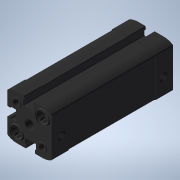
# Autodesk Inventor part: 537123 ADNGF-12-40-P-A---(Z)
Saved by Autodesk Inventor 2021 (Build 250183000, 183)
## iProperties
Created: 2025-06-05
Part Number: 537123 ADNGF-12-40-P-A---(Z)
Material: Generic
Catalog Web Link: www.cadenas.de
Description: ADN-(Z(mm))-Compact cylinder - Z
Vendor: FESTO
Document SubType Name: Modeling
Designer: psAdmin
Manufacturer: FESTO
Mass: 35.9868 g
Surface Area: 194.795 cm^2
Volume: 35.9868 cm^3
Density: 1 g/cm^3
Appearance: PSOLRGB-175-175-175
Category: PARTsolutions
Company: FESTO
Title: 537123 ADNGF-12-40-P-A---(Z)
Author: Cadenas PARTsolutions
Comments: Compact cylinder - Z
PSOL_IDENT_0: {$CADENAS_DATA/23d-libs/festo/parts/a/adngf/parts/adngf_zr.prj},215 {VTYP=3D},{NB=537123 ADNGF-12-40
PSOL_IDENT_1: -P-A---(Z)},{LINA=537123 ADNGF-12-40-P-A---(Z)},{NN=ADN-(Z(mm))},{DATE=02.05.2022 13:23:46},{GEOMDAT
PSOL_IDENT_2: E=06.10.2021 08:16:00},{VERSION=},{LINEID=5510},{WBVAR=HUB,S2S20},{WBNUMERIC=HUB}  {NB=537123 ADNGF-
PSOL_IDENT_3: 12-40-P-A---(Z)},{LINA=537123 ADNGF-12-40-P-A---(Z)},{KT=ADNGF-12},{TNR=537123},{AUSF=ADNGF-12},{KDM=
PSOL_IDENT_4: 12},{BG=17.000},{VERS=1},{HUB=40.00000},{HUB1=1.000},{HUB2=200.000},{ED=P-A},{Q=-},{S2S20=-},{S1=-},
PSOL_IDENT_5: {R8=-},{TT=-},{A=10.000},{A1=0.000},{AF=8.000},{AF1=0.000},{AF2=8.000},{AF3=0.000},{B=0.000},{B1=0.0
PSOL_IDENT_6: 00},{BG1=0.000},{D1=9.000},{D2=6.000},{D3=32.000},{D4=0.000},{D5=4.000},{D6=M3},{D7=3.000},{D8=0.000
PSOL_IDENT_7: },{D9=0.000},{E=27.500},{EE=M5},{EEN=5.000},{EE1=-},{J=10.500},{J1=2.000},{J11=2},{J2=0.000},{KF=4-4
PSOL_IDENT_8: 8 UNF-2B},{KF1=-},{KF2=4-45 UNF-2B},{KF3=-},{KK=10-32 UNF-2A},{KK1=-},{L1=1.500},{L2=35.000},{L3=2.1
PSOL_IDENT_9: 00},{L4=3.500},{L5=0.000},{L6=46.000},{L7=12.000},{L8=0.000},{L9=1.500},{L10=0.000},{L11=0.000},{MF=
PSOL_IDENT_10: 6.000},{MM=6.000},{MM1=0.000},{PL=6.000},{RT=M4},{RTN=4},{RTNK=3.242},{SF=3/16},{SF1=-},{SW=5.500},{
PSOL_IDENT_11: TG=16.000},{VD=0.000},{VD1=0.000},{WH=4.200},{WH1=0.000},{WL=2.700},{WL1=0.000},{Y1=0.300},{Y2=0.500
PSOL_IDENT_12: },{ZJ=39.200},{ZM=43.400},{RU=16.600},{R1=10.350},{R2=0.600},{RA=0.600},{RR=5.600},{RB1=5.400},{RB2=
PSOL_IDENT_13: 6.800},{RT1=3.400},{DSK=6.000},{MDK=5.500},{MK=3.000},{MT=1.300},{MS=2.500},{RUB=0.200},{KFN=3.000},
PSOL_IDENT_14: {KFK=2.459},{B111=9.200},{B11=1.000},{B2=5.000},{B3=8.500},{B4=3.500},{B5=3.000},{B6=6.000},{B7=17.0
PSOL_IDENT_15: 00},{B8=4.000},{B9=6.000},{B10=7.200},{W=0.400},{S=6.000},{LA=0.000},{LA1=0.000},{LA2=5.500},{LA3=7.
PSOL_IDENT_16: 000},{LA31=8.000},{LA4=0.000},{LA5=0.000},{LA6=0.000},{LA7=0.000},{LA8=0.000},{LA9=0.000},{LA10=0.00
PSOL_IDENT_17: 0},{ES=0.000},{SS=0.000},{TS=0.000},{WS=0.000},{DK=0.000},{KS=0.000},{S2N=},{D10=5.500},{D11=6.200},
PSOL_IDENT_18: {D12=0.200},{D13=4.000},{D14=0.000},{L12=15.000},{L13=4.200}
NB: 537123 ADNGF-12-40-P-A---(Z)
NN: ADN-(Z(mm))
NT: Compact cylinder - Z
NBSYN: $TNR. $AUSF.-$HUB.-$ED.$S2N.---(Z)
LINA: 537123 ADNGF-12-40-P-A---(Z)
CATALOG: Festo
TNR: 537123
AUSF: ADNGF-12
KDM: 12
BG: 17
HUB: 40
ED: P-A
Q: -
S2S20: -
S1: -
R8: -
TT: -
A: 10
A1: 0
AF: 8
AF1: 0
AF2: 8
AF3: 0
B: 0
B1: 0
BG1: 0
D1: 9
D2: 6
D3: 32
D4: 0
D5: 4
D6: M3
D7: 3
D8: 0
D9: 0
E: 27.5
EE: M5
EE1: -
J: 10.5
J1: 2
J2: 0
KF: 4-48 UNF-2B
KF1: -
KF2: 4-45 UNF-2B
KF3: -
KK: 10-32 UNF-2A
KK1: -
L1: 1.5
L2: 35
L3: 2.1
L4: 3.5
L5: 0
L6: 46
L7: 12
L8: 0
L9: 1.5
L10: 0
L11: 0
MF: 6
MM: 6
MM1: 0
PL: 6
RT: M4
RTNK: 3.242
SF: 3/16
SF1: -
SW: 5.5
TG: 16
VD: 0
VD1: 0
WH: 4.2
WH1: 0
WL: 2.7
WL1: 0
Y1: 0.3
Y2: 0.5
ZJ: 39.2
ZM: 43.4
RU: 16.6
R1: 10.35
R2: 0.6
RA: 0.6
RR: 5.6
DSK: 6
MDK: 5.5
MK: 3
MT: 1.3
MS: 2.5
RUB: 0.2
B111: 9.2
B11: 1
B2: 5
B3: 8.5
B4: 3.5
B5: 3
B6: 6
B7: 17
B8: 4
B9: 6
B10: 7.2
W: 0.4
S: 6
LA: 0
LA1: 0
LA2: 5.5
LA3: 7
LA31: 8
LA4: 0
LA5: 0
LA6: 0
LA7: 0
LA8: 0
LA9: 0
LA10: 0
ES: 0
SS: 0
TS: 0
WS: 0
DK: 0
KS: 0
D10: 5.5
D11: 6.2
D12: 0.2
D13: 4
D14: 0
L12: 15
L13: 4.2
SUPPLIER: FESTO
ARTICLENO: 537123 ADNGF-12-40-P-A---(Z)
BOMINFO: 537123 ADNGF-12-40-P-A---(Z)
CREATOR: CADENAS GmbH
Autodesk Inventor part; units mm, degrees
sketch "Sketch_26" plane through (0, 0, 0) normal (0, 0, 1) x (1, 0, 0)
  line L0 (-13.75, -2.5) -> (-13.75, -11.5793)
  arc A0 (-13.75, -11.5793) -> (-13.3272, -12.3141) centre (-12.9, -11.5793) ccw
  arc A1 (-13.3272, -12.3141) -> (-8, -13.75) centre (-8, -3.15) ccw
  line L1 (-8, -13.75) -> (-2.5, -13.75)
  arc A2 (-2.5, -13.75) -> (-2.1, -13.35) centre (-2.5, -13.35) ccw
  line L2 (-2.1, -13.35) -> (-2.1, -11.9)
  arc A3 (-2.1, -11.9) -> (-2.3, -11.7) centre (-2.3, -11.9) ccw
  line L3 (-2.3, -11.7) -> (-2.6, -11.7)
  arc A4 (-2.8, -11.5) -> (-2.6, -11.7) centre (-2.6, -11.5) ccw
  line L4 (-2.8, -11.5) -> (-2.8, -8.7)
  arc A5 (-2.4, -8.3) -> (-2.8, -8.7) centre (-2.4, -8.7) ccw
  line L5 (-2.4, -8.3) -> (3.6, -8.3)
  arc A6 (4, -8.7) -> (3.6, -8.3) centre (3.6, -8.7) ccw
  line L6 (4, -8.7) -> (4, -11.5)
  arc A7 (3.8, -11.7) -> (4, -11.5) centre (3.8, -11.5) ccw
  line L7 (3.8, -11.7) -> (3.5, -11.7)
  arc A8 (3.5, -11.7) -> (3.3, -11.9) centre (3.5, -11.9) ccw
  line L8 (3.3, -11.9) -> (3.3, -13.35)
  arc A9 (3.3, -13.35) -> (3.7, -13.75) centre (3.7, -13.35) ccw
  line L9 (3.7, -13.75) -> (8, -13.75)
  arc A10 (8, -13.75) -> (13.3272, -12.3141) centre (8, -3.15) ccw
  arc A11 (13.3272, -12.3141) -> (13.75, -11.5793) centre (12.9, -11.5793) ccw
  line L10 (13.75, -11.5793) -> (13.75, 11.5793)
  arc A12 (13.75, 11.5793) -> (13.3272, 12.3141) centre (12.9, 11.5793) ccw
  arc A13 (13.3272, 12.3141) -> (8, 13.75) centre (8, 3.15) ccw
  line L11 (8, 13.75) -> (2.5, 13.75)
  arc A14 (2.5, 13.75) -> (2.1, 13.35) centre (2.5, 13.35) ccw
  line L12 (2.1, 13.35) -> (2.1, 11.9)
  arc A15 (2.1, 11.9) -> (2.3, 11.7) centre (2.3, 11.9) ccw
  line L13 (2.3, 11.7) -> (2.6, 11.7)
  arc A16 (2.8, 11.5) -> (2.6, 11.7) centre (2.6, 11.5) ccw
  line L14 (2.8, 11.5) -> (2.8, 8.7)
  arc A17 (2.4, 8.3) -> (2.8, 8.7) centre (2.4, 8.7) ccw
  line L15 (2.4, 8.3) -> (-3.6, 8.3)
  arc A18 (-4, 8.7) -> (-3.6, 8.3) centre (-3.6, 8.7) ccw
  line L16 (-4, 8.7) -> (-4, 11.5)
  arc A19 (-3.8, 11.7) -> (-4, 11.5) centre (-3.8, 11.5) ccw
  line L17 (-3.8, 11.7) -> (-3.5, 11.7)
  arc A20 (-3.5, 11.7) -> (-3.3, 11.9) centre (-3.5, 11.9) ccw
  line L18 (-3.3, 11.9) -> (-3.3, 13.35)
  arc A21 (-3.3, 13.35) -> (-3.7, 13.75) centre (-3.7, 13.35) ccw
  line L19 (-3.7, 13.75) -> (-8, 13.75)
  arc A22 (-8, 13.75) -> (-13.3272, 12.3141) centre (-8, 3.15) ccw
  arc A23 (-13.3272, 12.3141) -> (-13.75, 11.5793) centre (-12.9, 11.5793) ccw
  line L20 (-13.75, 11.5793) -> (-13.75, 3.7)
  arc A24 (-13.75, 3.7) -> (-13.35, 3.3) centre (-13.35, 3.7) ccw
  line L21 (-13.35, 3.3) -> (-11.9, 3.3)
  arc A25 (-11.9, 3.3) -> (-11.7, 3.5) centre (-11.9, 3.5) ccw
  line L22 (-11.7, 3.5) -> (-11.7, 3.8)
  arc A26 (-11.5, 4) -> (-11.7, 3.8) centre (-11.5, 3.8) ccw
  line L23 (-11.5, 4) -> (-8.7, 4)
  arc A27 (-8.3, 3.6) -> (-8.7, 4) centre (-8.7, 3.6) ccw
  line L24 (-8.3, 3.6) -> (-8.3, -2.4)
  arc A28 (-8.7, -2.8) -> (-8.3, -2.4) centre (-8.7, -2.4) ccw
  line L25 (-8.7, -2.8) -> (-11.5, -2.8)
  arc A29 (-11.7, -2.6) -> (-11.5, -2.8) centre (-11.5, -2.6) ccw
  line L26 (-11.7, -2.6) -> (-11.7, -2.3)
  arc A30 (-11.7, -2.3) -> (-11.9, -2.1) centre (-11.9, -2.3) ccw
  line L27 (-11.9, -2.1) -> (-13.35, -2.1)
  arc A31 (-13.35, -2.1) -> (-13.75, -2.5) centre (-13.35, -2.5) ccw
  constraints: 64 point on circle, 56 end point, 32 centre point
extrude "Extrusion1" add sketch "Sketch_26" against normal blind 75
sketch "Sketch_112" plane through (0, 0, -10.5) normal (0, 0, 1) x (1, 0, 0)
  line L0 (-27.5, -27.5) -> (27.5, -27.5)
  line L1 (27.5, -27.5) -> (27.5, 27.5)
  line L2 (27.5, 27.5) -> (-27.5, 27.5)
  line L3 (-27.5, 27.5) -> (-27.5, -27.5)
  line L4 (-13.5, -2.5) -> (-13.5, -11.3293)
  arc A0 (-13.5, -11.3293) -> (-13.0772, -12.0641) centre (-12.65, -11.3293) ccw
  arc A1 (-13.0772, -12.0641) -> (-7.75, -13.5) centre (-7.75, -2.9) ccw
  line L5 (-7.75, -13.5) -> (-2.5, -13.5)
  arc A2 (-2.5, -13.5) -> (-2.1, -13.1) centre (-2.5, -13.1) ccw
  line L6 (-2.1, -13.1) -> (-2.1, -11.9)
  arc A3 (-2.1, -11.9) -> (-2.3, -11.7) centre (-2.3, -11.9) ccw
  line L7 (-2.3, -11.7) -> (-2.6, -11.7)
  arc A4 (-2.8, -11.5) -> (-2.6, -11.7) centre (-2.6, -11.5) ccw
  line L8 (-2.8, -11.5) -> (-2.8, -8.7)
  arc A5 (-2.4, -8.3) -> (-2.8, -8.7) centre (-2.4, -8.7) ccw
  line L9 (-2.4, -8.3) -> (3.6, -8.3)
  arc A6 (4, -8.7) -> (3.6, -8.3) centre (3.6, -8.7) ccw
  line L10 (4, -8.7) -> (4, -11.5)
  arc A7 (3.8, -11.7) -> (4, -11.5) centre (3.8, -11.5) ccw
  line L11 (3.8, -11.7) -> (3.5, -11.7)
  arc A8 (3.5, -11.7) -> (3.3, -11.9) centre (3.5, -11.9) ccw
  line L12 (3.3, -11.9) -> (3.3, -13.1)
  arc A9 (3.3, -13.1) -> (3.7, -13.5) centre (3.7, -13.1) ccw
  line L13 (3.7, -13.5) -> (7.75, -13.5)
  arc A10 (7.75, -13.5) -> (13.0772, -12.0641) centre (7.75, -2.9) ccw
  arc A11 (13.0772, -12.0641) -> (13.5, -11.3293) centre (12.65, -11.3293) ccw
  line L14 (13.5, -11.3293) -> (13.5, 11.3293)
  arc A12 (13.5, 11.3293) -> (13.0772, 12.0641) centre (12.65, 11.3293) ccw
  arc A13 (13.0772, 12.0641) -> (7.75, 13.5) centre (7.75, 2.9) ccw
  line L15 (7.75, 13.5) -> (2.5, 13.5)
  arc A14 (2.5, 13.5) -> (2.1, 13.1) centre (2.5, 13.1) ccw
  line L16 (2.1, 13.1) -> (2.1, 11.9)
  arc A15 (2.1, 11.9) -> (2.3, 11.7) centre (2.3, 11.9) ccw
  line L17 (2.3, 11.7) -> (2.6, 11.7)
  arc A16 (2.8, 11.5) -> (2.6, 11.7) centre (2.6, 11.5) ccw
  line L18 (2.8, 11.5) -> (2.8, 8.7)
  arc A17 (2.4, 8.3) -> (2.8, 8.7) centre (2.4, 8.7) ccw
  line L19 (2.4, 8.3) -> (-3.6, 8.3)
  arc A18 (-4, 8.7) -> (-3.6, 8.3) centre (-3.6, 8.7) ccw
  line L20 (-4, 8.7) -> (-4, 11.5)
  arc A19 (-3.8, 11.7) -> (-4, 11.5) centre (-3.8, 11.5) ccw
  line L21 (-3.8, 11.7) -> (-3.5, 11.7)
  arc A20 (-3.5, 11.7) -> (-3.3, 11.9) centre (-3.5, 11.9) ccw
  line L22 (-3.3, 11.9) -> (-3.3, 13.1)
  arc A21 (-3.3, 13.1) -> (-3.7, 13.5) centre (-3.7, 13.1) ccw
  line L23 (-3.7, 13.5) -> (-7.75, 13.5)
  arc A22 (-7.75, 13.5) -> (-13.0772, 12.0641) centre (-7.75, 2.9) ccw
  arc A23 (-13.0772, 12.0641) -> (-13.5, 11.3293) centre (-12.65, 11.3293) ccw
  line L24 (-13.5, 11.3293) -> (-13.5, 3.7)
  arc A24 (-13.5, 3.7) -> (-13.1, 3.3) centre (-13.1, 3.7) ccw
  line L25 (-13.1, 3.3) -> (-11.9, 3.3)
  arc A25 (-11.9, 3.3) -> (-11.7, 3.5) centre (-11.9, 3.5) ccw
  line L26 (-11.7, 3.5) -> (-11.7, 3.8)
  arc A26 (-11.5, 4) -> (-11.7, 3.8) centre (-11.5, 3.8) ccw
  line L27 (-11.5, 4) -> (-8.7, 4)
  arc A27 (-8.3, 3.6) -> (-8.7, 4) centre (-8.7, 3.6) ccw
  line L28 (-8.3, 3.6) -> (-8.3, -2.4)
  arc A28 (-8.7, -2.8) -> (-8.3, -2.4) centre (-8.7, -2.4) ccw
  line L29 (-8.7, -2.8) -> (-11.5, -2.8)
  arc A29 (-11.7, -2.6) -> (-11.5, -2.8) centre (-11.5, -2.6) ccw
  line L30 (-11.7, -2.6) -> (-11.7, -2.3)
  arc A30 (-11.7, -2.3) -> (-11.9, -2.1) centre (-11.9, -2.3) ccw
  line L31 (-11.9, -2.1) -> (-13.1, -2.1)
  arc A31 (-13.1, -2.1) -> (-13.5, -2.5) centre (-13.1, -2.5) ccw
  constraints: 64 end point, 64 point on circle, 32 centre point
extrude "Extrusion2" cut sketch "Sketch_112" against normal blind 54
sketch "Sketch3" plane through (13.75, -11.5793, 0) normal (1, 0, 0) x (0, 0, -1)
  point P0 (6, 9.5793)
hole "Hole1" at (13.75, -2, -6) direction (-1, 0, 0) diameter 4.134 depth 7 countersink diameter 5 countersink angle 90 thread size "M5x0.8" class "6H" standard "ISO Metric profile"
sketch "Sketch4" plane through (13.75, -11.5793, -75) normal (1, 0, 0) x (0, 0, -1)
  point P0 (-6, 9.5793)
hole "Hole2" at (13.75, -2, -69) direction (-1, 0, 0) diameter 4.134 depth 8 countersink diameter 5 countersink angle 90 thread size "M5x0.8" class "6H" standard "ISO Metric profile"
sketch "Skizze_5" plane through (0, 0, 0) normal (1, 0, 0) x (0, 1, 0)
  line L0 (0, -63) -> (0, 1)
  line L1 (0, 1) -> (3, 1)
  line L2 (3, 1) -> (3, -20)
  line L3 (3, -20) -> (6, -20)
  line L4 (6, -20) -> (6, -63)
  line L5 (6, -63) -> (0, -63)
  line L6 (0, -63) -> (0, 1)
  constraints: 14 end point
revolve "Revolution1" cut sketch "Skizze_5" angle 360 about axis through (0, 0, -63) along (0, 0, -1)
sketch "Sketch6" plane through (0, 0, -75) normal (0, 0, -1) x (-1, 0, 0)
  point P0 (0, 0)
hole "Hole3" at (0, 0, -75) direction (0, 0, 1) diameter 9 depth 2.1
sketch "Sketch7" plane through (0, 0, 0) normal (0, 0, 1) x (1, 0, 0)
  point P0 (8, 8)
hole "Hole4" at (8, 8, 0) direction (0, 0, -1) diameter 6 depth 17 counterbore diameter 9.2 counterbore depth 5
sketch "Sketch_27" plane through (8, 0, 0) normal (1, 0, 0) x (0, 0, -1)
  line L0 (17, 8) -> (0, 8)
  line L1 (0, 11.6) -> (1.0392, 11)
  line L2 (1.0392, 11) -> (3.5, 11)
  line L3 (3.5, 11) -> (3.5, 10)
  line L4 (3.5, 10) -> (3.879, 9.621)
  line L5 (3.879, 9.621) -> (17, 9.621)
  line L6 (17, 9.621) -> (17, 12)
  line L7 (17, 12) -> (5, 12)
  line L8 (5, 12) -> (5, 12.25)
  line L9 (5, 12.25) -> (0.4, 12.25)
  line L10 (0.4, 12.25) -> (0, 11.85)
  line L11 (0, 11.85) -> (0, 11.6)
  constraints: 24 end point
revolve "Revolution2" add sketch "Sketch_27" angle 360 about axis through (8, 8, -17) along (0, 0, -1)
thread "Thread1" size "M4x0.7" class "6H" standard "ISO Metric profile" full length
sketch "Sketch9" plane through (0, 0, -75) normal (0, 0, -1) x (-1, 0, 0)
  point P0 (-8, 8)
hole "Hole5" at (8, 8, -75) direction (0, 0, 1) diameter 6 depth 17 counterbore diameter 9.2 counterbore depth 5
sketch "Sketch10" plane through (8, 8, -58) normal (0, 0, -1) x (-1, 0, 0)
  point P0 (0, 0)
hole "Hole6" at (8, 8, -58) direction (0, 0, 1) diameter 5.6 depth 41
sketch "Sketch_28" plane through (8, 0, 0) normal (1, 0, 0) x (0, 0, -1)
  line L0 (75, 8) -> (58, 8)
  line L1 (58, 12) -> (58, 9.621)
  line L2 (58, 9.621) -> (71.121, 9.621)
  line L3 (71.121, 9.621) -> (71.5, 10)
  line L4 (71.5, 10) -> (71.5, 11)
  line L5 (71.5, 11) -> (73.9608, 11)
  line L6 (73.9608, 11) -> (75, 11.6)
  line L7 (75, 11.6) -> (75, 11.85)
  line L8 (75, 11.85) -> (74.6, 12.25)
  line L9 (74.6, 12.25) -> (70, 12.25)
  line L10 (70, 12.25) -> (70, 12)
  line L11 (70, 12) -> (58, 12)
  constraints: 24 end point
revolve "Revolution3" add sketch "Sketch_28" angle 360 about axis through (8, 8, -75) along (0, 0, -1)
thread "Thread2" size "M4x0.7" class "6H" standard "ISO Metric profile" full length
sketch "Sketch12" plane through (0, 0, 0) normal (0, 0, 1) x (1, 0, 0)
  point P0 (-8, -8)
hole "Hole7" at (-8, -8, 0) direction (0, 0, -1) diameter 6 depth 17 counterbore diameter 9.2 counterbore depth 5
sketch "Sketch13" plane through (0, 0, -75) normal (0, 0, -1) x (-1, 0, 0)
  point P0 (8, -8)
hole "Hole8" at (-8, -8, -75) direction (0, 0, 1) diameter 6 depth 17 counterbore diameter 9.2 counterbore depth 5
sketch "Sketch_29" plane through (-8, 0, 0) normal (1, 0, 0) x (0, 0, -1)
  line L0 (17, -8) -> (0, -8)
  line L1 (0, -4.4) -> (1.0392, -5)
  line L2 (1.0392, -5) -> (3.5, -5)
  line L3 (3.5, -5) -> (3.5, -6)
  line L4 (3.5, -6) -> (3.879, -6.379)
  line L5 (3.879, -6.379) -> (17, -6.379)
  line L6 (17, -6.379) -> (17, -4)
  line L7 (17, -4) -> (5, -4)
  line L8 (5, -4) -> (5, -3.75)
  line L9 (5, -3.75) -> (0.4, -3.75)
  line L10 (0.4, -3.75) -> (0, -4.15)
  line L11 (0, -4.15) -> (0, -4.4)
  constraints: 24 end point
revolve "Revolution4" add sketch "Sketch_29" angle 360 about axis through (-8, -8, -17) along (0, 0, -1)
thread "Thread3" size "M4x0.7" class "6H" standard "ISO Metric profile" full length
sketch "Sketch_30" plane through (-8, 0, 0) normal (1, 0, 0) x (0, 0, -1)
  line L0 (75, -8) -> (58, -8)
  line L1 (58, -4) -> (58, -6.379)
  line L2 (58, -6.379) -> (71.121, -6.379)
  line L3 (71.121, -6.379) -> (71.5, -6)
  line L4 (71.5, -6) -> (71.5, -5)
  line L5 (71.5, -5) -> (73.9608, -5)
  line L6 (73.9608, -5) -> (75, -4.4)
  line L7 (75, -4.4) -> (75, -4.15)
  line L8 (75, -4.15) -> (74.6, -3.75)
  line L9 (74.6, -3.75) -> (70, -3.75)
  line L10 (70, -3.75) -> (70, -4)
  line L11 (70, -4) -> (58, -4)
  constraints: 24 end point
revolve "Revolution5" add sketch "Sketch_30" angle 360 about axis through (-8, -8, -75) along (0, 0, -1)
thread "Thread4" size "M4x0.7" class "6H" standard "ISO Metric profile" full length
sketch "Sketch16" plane through (0, 0, 0) normal (0, 0, 1) x (1, 0, 0)
  point P0 (8, -8)
hole "Hole9" at (8, -8, 0) direction (0, 0, -1) diameter 4 depth 58 counterbore diameter 5.5 counterbore depth 10.5
sketch "Sketch_14" plane through (8, 0, 0) normal (1, 0, 0) x (0, 0, -1)
  line L0 (14.7, -8) -> (-0.3, -8)
  line L1 (-0.3, -6) -> (14.7, -6)
  line L2 (14.7, -6) -> (14.7, -4.9)
  line L3 (14.7, -4.9) -> (10.5, -4.9)
  line L4 (10.5, -4.9) -> (10.5, -5.25)
  line L5 (10.5, -5.25) -> (-0.1, -5.25)
  line L6 (-0.1, -5.25) -> (-0.3, -5.3655)
  line L7 (-0.3, -5.3655) -> (-0.3, -6)
  constraints: 16 end point
revolve "Revolution6" add sketch "Sketch_14" angle 360 about axis through (8, -8, -14.7) along (0, 0, -1)
sketch "Sketch_3" plane through (8, 0, 0) normal (1, 0, 0) x (0, 0, -1)
  line L0 (75.1, -8) -> (64.5, -8)
  line L1 (64.5, -8) -> (64.5, -6.379)
  line L2 (64.5, -6.379) -> (71.121, -6.379)
  line L3 (71.121, -6.379) -> (71.5, -6)
  line L4 (71.5, -6) -> (71.5, -5)
  line L5 (71.5, -5) -> (75.1, -5)
  line L6 (75.1, -5) -> (75.1, -8)
  line L7 (75.1, -8) -> (64.5, -8)
  constraints: 16 end point
revolve "Revolution7" cut sketch "Sketch_3" angle 360 about axis through (8, -8, -75.1) along (0, 0, -1)
thread "Thread5" size "M4x0.7" class "6H" standard "ISO Metric profile" full length
sketch "Sketch19" plane through (8, -8, -64.5) normal (0, 0, -1) x (-1, 0, 0)
  point P0 (0, 0)
hole "Hole10" at (8, -8, -64.5) direction (0, 0, 1) diameter 4 depth 47.5
sketch "Sketch20" plane through (0, 0, 0) normal (0, 0, 1) x (1, 0, 0)
  point P0 (-8, 8)
hole "Hole11" at (-8, 8, 0) direction (0, 0, -1) diameter 4 depth 58 counterbore diameter 5.5 counterbore depth 10.5
sketch "Sketch_15" plane through (-8, 0, 0) normal (1, 0, 0) x (0, 0, -1)
  line L0 (14.7, 8) -> (-0.3, 8)
  line L1 (-0.3, 10) -> (14.7, 10)
  line L2 (14.7, 10) -> (14.7, 11.1)
  line L3 (14.7, 11.1) -> (10.5, 11.1)
  line L4 (10.5, 11.1) -> (10.5, 10.75)
  line L5 (10.5, 10.75) -> (-0.1, 10.75)
  line L6 (-0.1, 10.75) -> (-0.3, 10.6345)
  line L7 (-0.3, 10.6345) -> (-0.3, 10)
  constraints: 16 end point
revolve "Revolution8" add sketch "Sketch_15" angle 360 about axis through (-8, 8, -14.7) along (0, 0, -1)
sketch "Sketch_4" plane through (-8, 0, 0) normal (1, 0, 0) x (0, 0, -1)
  line L0 (75.1, 8) -> (64.5, 8)
  line L1 (64.5, 8) -> (64.5, 9.621)
  line L2 (64.5, 9.621) -> (71.121, 9.621)
  line L3 (71.121, 9.621) -> (71.5, 10)
  line L4 (71.5, 10) -> (71.5, 11)
  line L5 (71.5, 11) -> (75.1, 11)
  line L6 (75.1, 11) -> (75.1, 8)
  line L7 (75.1, 8) -> (64.5, 8)
  constraints: 16 end point
revolve "Revolution9" cut sketch "Sketch_4" angle 360 about axis through (-8, 8, -75.1) along (0, 0, -1)
thread "Thread6" size "M4x0.7" class "6H" standard "ISO Metric profile" full length
sketch "Sketch23" plane through (-8, 8, -64.5) normal (0, 0, -1) x (-1, 0, 0)
  point P0 (0, 0)
hole "Hole12" at (-8, 8, -64.5) direction (0, 0, 1) diameter 4 depth 47.5
sketch "Sketch24" plane through (-8, -8, -58) normal (0, 0, -1) x (-1, 0, 0)
  point P0 (0, 0)
hole "Hole13" at (-8, -8, -58) direction (0, 0, 1) diameter 5.6 depth 41
sketch "Sketch_8" plane through (0, 0, 0) normal (0, 0, 1) x (1, 0, 0)
  line L0 (-11.4641, -8) -> (-11, -8.8038)
  line L1 (-11, -8.8038) -> (-11, -9.7321)
  line L2 (-11, -9.7321) -> (-10.1962, -10.1962)
  line L3 (-10.1962, -10.1962) -> (-9.7321, -11)
  line L4 (-9.7321, -11) -> (-8.8038, -11)
  line L5 (-8.8038, -11) -> (-8, -11.4641)
  line L6 (-8, -11.4641) -> (-7.1962, -11)
  line L7 (-7.1962, -11) -> (-6.2679, -11)
  line L8 (-6.2679, -11) -> (-5.8038, -10.1962)
  line L9 (-5.8038, -10.1962) -> (-5, -9.7321)
  line L10 (-5, -9.7321) -> (-5, -8.8038)
  line L11 (-5, -8.8038) -> (-4.5359, -8)
  line L12 (-4.5359, -8) -> (-5, -7.1962)
  line L13 (-5, -7.1962) -> (-5, -6.2679)
  line L14 (-5, -6.2679) -> (-5.8038, -5.8038)
  line L15 (-5.8038, -5.8038) -> (-6.2679, -5)
  line L16 (-6.2679, -5) -> (-7.1962, -5)
  line L17 (-7.1962, -5) -> (-8, -4.5359)
  line L18 (-8, -4.5359) -> (-8.8038, -5)
  line L19 (-8.8038, -5) -> (-9.7321, -5)
  line L20 (-9.7321, -5) -> (-10.1962, -5.8038)
  line L21 (-10.1962, -5.8038) -> (-11, -6.2679)
  line L22 (-11, -6.2679) -> (-11, -7.1962)
  line L23 (-11, -7.1962) -> (-11.4641, -8)
  constraints: 48 end point
extrude "Extrusion3" cut sketch "Sketch_8" against normal blind 3
sketch "Sketch_7" plane through (0, 0, 0) normal (0, 0, 1) x (1, 0, 0)
  line L0 (4.5359, 8) -> (5, 7.1962)
  line L1 (5, 7.1962) -> (5, 6.2679)
  line L2 (5, 6.2679) -> (5.8038, 5.8038)
  line L3 (5.8038, 5.8038) -> (6.2679, 5)
  line L4 (6.2679, 5) -> (7.1962, 5)
  line L5 (7.1962, 5) -> (8, 4.5359)
  line L6 (8, 4.5359) -> (8.8038, 5)
  line L7 (8.8038, 5) -> (9.7321, 5)
  line L8 (9.7321, 5) -> (10.1962, 5.8038)
  line L9 (10.1962, 5.8038) -> (11, 6.2679)
  line L10 (11, 6.2679) -> (11, 7.1962)
  line L11 (11, 7.1962) -> (11.4641, 8)
  line L12 (11.4641, 8) -> (11, 8.8038)
  line L13 (11, 8.8038) -> (11, 9.7321)
  line L14 (11, 9.7321) -> (10.1962, 10.1962)
  line L15 (10.1962, 10.1962) -> (9.7321, 11)
  line L16 (9.7321, 11) -> (8.8038, 11)
  line L17 (8.8038, 11) -> (8, 11.4641)
  line L18 (8, 11.4641) -> (7.1962, 11)
  line L19 (7.1962, 11) -> (6.2679, 11)
  line L20 (6.2679, 11) -> (5.8038, 10.1962)
  line L21 (5.8038, 10.1962) -> (5, 9.7321)
  line L22 (5, 9.7321) -> (5, 8.8038)
  line L23 (5, 8.8038) -> (4.5359, 8)
  constraints: 48 end point
extrude "Extrusion4" cut sketch "Sketch_7" against normal blind 3
sketch "Sketch_9" plane through (0, 0, -75) normal (0, 0, 1) x (1, 0, 0)
  line L0 (-11.4641, -8) -> (-11, -8.8038)
  line L1 (-11, -8.8038) -> (-11, -9.7321)
  line L2 (-11, -9.7321) -> (-10.1962, -10.1962)
  line L3 (-10.1962, -10.1962) -> (-9.7321, -11)
  line L4 (-9.7321, -11) -> (-8.8038, -11)
  line L5 (-8.8038, -11) -> (-8, -11.4641)
  line L6 (-8, -11.4641) -> (-7.1962, -11)
  line L7 (-7.1962, -11) -> (-6.2679, -11)
  line L8 (-6.2679, -11) -> (-5.8038, -10.1962)
  line L9 (-5.8038, -10.1962) -> (-5, -9.7321)
  line L10 (-5, -9.7321) -> (-5, -8.8038)
  line L11 (-5, -8.8038) -> (-4.5359, -8)
  line L12 (-4.5359, -8) -> (-5, -7.1962)
  line L13 (-5, -7.1962) -> (-5, -6.2679)
  line L14 (-5, -6.2679) -> (-5.8038, -5.8038)
  line L15 (-5.8038, -5.8038) -> (-6.2679, -5)
  line L16 (-6.2679, -5) -> (-7.1962, -5)
  line L17 (-7.1962, -5) -> (-8, -4.5359)
  line L18 (-8, -4.5359) -> (-8.8038, -5)
  line L19 (-8.8038, -5) -> (-9.7321, -5)
  line L20 (-9.7321, -5) -> (-10.1962, -5.8038)
  line L21 (-10.1962, -5.8038) -> (-11, -6.2679)
  line L22 (-11, -6.2679) -> (-11, -7.1962)
  line L23 (-11, -7.1962) -> (-11.4641, -8)
  constraints: 48 end point
extrude "Extrusion5" cut sketch "Sketch_9" along normal blind 3
sketch "Sketch_10" plane through (0, 0, -75) normal (0, 0, 1) x (1, 0, 0)
  line L0 (4.5359, 8) -> (5, 7.1962)
  line L1 (5, 7.1962) -> (5, 6.2679)
  line L2 (5, 6.2679) -> (5.8038, 5.8038)
  line L3 (5.8038, 5.8038) -> (6.2679, 5)
  line L4 (6.2679, 5) -> (7.1962, 5)
  line L5 (7.1962, 5) -> (8, 4.5359)
  line L6 (8, 4.5359) -> (8.8038, 5)
  line L7 (8.8038, 5) -> (9.7321, 5)
  line L8 (9.7321, 5) -> (10.1962, 5.8038)
  line L9 (10.1962, 5.8038) -> (11, 6.2679)
  line L10 (11, 6.2679) -> (11, 7.1962)
  line L11 (11, 7.1962) -> (11.4641, 8)
  line L12 (11.4641, 8) -> (11, 8.8038)
  line L13 (11, 8.8038) -> (11, 9.7321)
  line L14 (11, 9.7321) -> (10.1962, 10.1962)
  line L15 (10.1962, 10.1962) -> (9.7321, 11)
  line L16 (9.7321, 11) -> (8.8038, 11)
  line L17 (8.8038, 11) -> (8, 11.4641)
  line L18 (8, 11.4641) -> (7.1962, 11)
  line L19 (7.1962, 11) -> (6.2679, 11)
  line L20 (6.2679, 11) -> (5.8038, 10.1962)
  line L21 (5.8038, 10.1962) -> (5, 9.7321)
  line L22 (5, 9.7321) -> (5, 8.8038)
  line L23 (5, 8.8038) -> (4.5359, 8)
  constraints: 48 end point
extrude "Extrusion6" cut sketch "Sketch_10" along normal blind 3
ref_plane "CYLINDER_XY" through (0, 0, -63) normal (0, 0, 1) x (1, 0, 0)
ref_plane "CYLINDER_YZ" through (0, 0, -63) normal (1, 0, 0) x (0, 1, 0)
ref_plane "CYLINDER_ZX" through (0, 0, -63) normal (0, 1, 0) x (0, 0, 1)
ref_plane "QS_HINTEN_XY" through (13.75, -2, -69) normal (1, 0, 0) x (0, 0, -1)
ref_plane "QS_HINTEN_YZ" through (13.75, -2, -69) normal (0, 0, -1) x (0, 1, 0)
ref_plane "QS_HINTEN_ZX" through (13.75, -2, -69) normal (0, 1, 0) x (1, 0, 0)
ref_plane "QS_VORNE_XY" through (13.75, -2, -6) normal (1, 0, 0) x (0, 0, -1)
ref_plane "QS_VORNE_YZ" through (13.75, -2, -6) normal (0, 0, -1) x (0, 1, 0)
ref_plane "QS_VORNE_ZX" through (13.75, -2, -6) normal (0, 1, 0) x (1, 0, 0)
ref_plane "TO_DUMMY_XY" through (0, 0, 0) normal (0, 0, 1) x (1, 0, 0)
ref_plane "TO_DUMMY_YZ" through (0, 0, 0) normal (1, 0, 0) x (0, 1, 0)
ref_plane "TO_DUMMY_ZX" through (0, 0, 0) normal (0, 1, 0) x (0, 0, 1)
ref_plane "ZUBEHOER_HINTEN_XY" through (0, 0, -75) normal (0, 0, 1) x (1, 0, 0)
ref_plane "ZUBEHOER_HINTEN_YZ" through (0, 0, -75) normal (1, 0, 0) x (0, 1, 0)
ref_plane "ZUBEHOER_HINTEN_ZX" through (0, 0, -75) normal (0, 1, 0) x (0, 0, 1)
ref_plane "ZUBEHOER_VORN_XY" through (0, 0, 0) normal (0, 0, 1) x (1, 0, 0)
ref_plane "ZUBEHOER_VORN_YZ" through (0, 0, 0) normal (1, 0, 0) x (0, 1, 0)
ref_plane "ZUBEHOER_VORN_ZX" through (0, 0, 0) normal (0, 1, 0) x (0, 0, 1)
body "Solid1"
